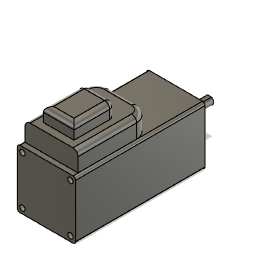
NEMA 23 Integrated Easy Servo Motor 130w v2 (Autodesk Fusion 360 design; units mm, degrees)
Autodesk Fusion 360 part; units mm, degrees
sketch "Sketch1" plane through (0, 0, 0) normal (0, 0, 1) x (1, 0, 0)
  line L0 (0, 0) -> (57.15, 0)
  line L1 (57.15, 0) -> (57.15, 57.15)
  line L2 (57.15, 57.15) -> (0, 57.15)
  line L3 (0, 57.15) -> (0, 0)
  circle A0 centre (52.125, 52.125) radius 2.6
  line L4 (28.575, 0) -> (28.575, 57.15) construction
  line L5 (0, 28.575) -> (57.15, 28.575) construction
  circle A1 centre (5.025, 52.125) radius 2.6
  circle A2 centre (5.025, 5.025) radius 2.6
  circle A3 centre (52.125, 5.025) radius 2.6
  circle A4 centre (28.575, 28.575) radius 19.05
  line L6 (2.575, 57.15) -> (54.575, 57.15)
  line L7 (54.575, 57.15) -> (54.575, 76)
  line L8 (54.575, 76) -> (2.575, 76)
  line L9 (2.575, 76) -> (2.575, 57.15)
  circle A5 centre (28.575, 28.575) radius 4
  line L10 (26.6385, 32.075) -> (30.5115, 32.075)
  line L11 (13.575, 76) -> (43.575, 76)
  line L12 (43.575, 76) -> (43.575, 89.67)
  line L13 (43.575, 89.67) -> (13.575, 89.67)
  line L14 (13.575, 89.67) -> (13.575, 76)
  point P0 (47.5479, 45.3005)
  dimension "d1" = 57.15
  dimension "d2" = 57.15
  dimension "d3" = 5.2
  dimension "d5" = 5.2
  dimension "d6" = 47.1
  dimension "d8" = 5.2
  dimension "d10" = 47.1
  dimension "d12" = 5.2
  dimension "d13" = 47.1
  dimension "d14" = 47.1
  dimension "d15" = 38.1
  dimension "d16" = 76
  dimension "d17" = 8
  dimension "d19" = 3.5
  dimension "d20" = 52
  dimension "d21" = 13.67
  dimension "d22" = 30
  constraint horizontal L0
  constraint vertical L1
  constraint horizontal L2
  constraint vertical L3
  constraint coincident L0.start L3.end
  constraint midpoint L0 L4.start
  constraint midpoint L2 L4.end
  constraint midpoint L3 L5.start
  constraint midpoint L1 L5.end
  constraint symmetric A0 L4 A1
  constraint symmetric L5 A1.centre A2.centre
  constraint midpoint L5 A4.centre
  constraint horizontal L6
  constraint vertical L7
  constraint horizontal L8
  constraint vertical L9
  constraint coincident L2 L6.start
  constraint concentric A4 A5
  constraint coincident A5 L10.start
  constraint coincident A5 L10.end
  constraint perpendicular L4 L10
  constraint symmetric L4 L7 L9
  constraint horizontal L11
  constraint vertical L12
  constraint horizontal L13
  constraint vertical L14
  constraint coincident L8 L11.start
  constraint symmetric L4 L12 L14
  measures "d1" distance of L0.start L0.end
  measures "d2" distance of L0.start L2.end
  measures "d3" diameter of A0
  measures "d5" diameter of A1
  measures "d6" distance of A0.centre A1.centre
  measures "d8" diameter of A2
  measures "d10" distance of A1.centre A2.centre
  measures "d12" diameter of A3
  measures "d13" horizontal distance of A2.centre A3.centre
  measures "d14" distance of A0.centre A3.centre
  measures "d15" diameter of A4
  measures "d16" distance of L0 L8
  measures "d17" diameter of A5
  measures "d19" distance of L5 L10
  measures "d20" distance of L7.end L8.end
  measures "d21" distance of L11.start L13.end
  measures "d22" distance of L12.end L13.end
extrude "Extrude1" add sketch "Sketch1" along normal blind 127 contours L0 L1 L2 L3 L6 | A4 | A5 L10 | A5 L10
fillet "Fillet1" radius 2.5 4 edges at (57.15, 57.15, 63.5) (57.15, 0, 63.5) (0, 0, 63.5) (0, 57.15, 63.5)
extrude "Extrude2" add sketch "Sketch1" against normal blind 70 from surface at 122 contours L2 L6 L7 L8 L9 L11
fillet "Fillet2" radius 12.5 2 edges at (54.575, 66.575, 52) (2.575, 66.575, 52)
fillet "Fillet2" radius 5 3 edges at (54.575, 76, 87) (28.575, 76, 52) (2.575, 76, 87)
extrude "Extrude3" add sketch "Sketch1" along normal blind 40 from surface at 75 contours L8 L11 L12 L13 L14
fillet "Fillet3" radius 5 6 edges at (43.575, 89.67, 95) (43.575, 82.835, 75) (13.575, 82.835, 75) (28.575, 89.67, 75) (13.575, 89.67, 95) (28.575, 89.67, 115)
extrude "Extrude4" add sketch "Sketch1" against normal blind 2 contours A4 | A5 L10 | A5 L10
extrude "Extrude5" add sketch "Sketch1" against normal blind 33 contours A5 L10 picked at (29.5161, 29.5962)
extrude "Extrude6" add sketch "Sketch1" against normal blind 6 contours A5 L10 picked at (28.1041, 32.1557)
equation "d10 = d6"
equation "d12 = d3"
equation "d13 = d6"
equation "d14 = d6"
equation "d19 = 7.5 mm - ( d17 / 2 )"
equation "d44 = ( -1 * ( 33 - 27 ) ) * 1 mm"
